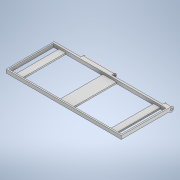
# Autodesk Inventor part: roof
Saved by Autodesk Inventor 2021 (Build 250183000, 183)
## iProperties
Created: 2021-08-17
Part Number: roof
Material: Generisch
Document SubType Name: Modeling
Designer: Tilman
Density: 1 g/cm^3
Appearance: Vorgabe
Author: Tilman
Autodesk Inventor part; units mm, degrees
ref_plane "YZ Plane" through (0, 0, 0) normal (1, 0, 0) x (0, 1, 0)
ref_plane "XZ Plane" through (0, 0, 0) normal (0, 1, 0) x (-1, 0, 0)
ref_plane "XY Plane" through (0, 0, 0) normal (0, 0, 1) x (1, 0, 0)
sketch "Skizze1" plane through (0, 0, 0) normal (0, 1, 0) x (-1, 0, 0)
  line L0 (0, 0) -> (-170, 0)
  line L1 (-170, 0) -> (-170, -70)
  line L2 (-170, -70) -> (0, -70)
  line L3 (0, -70) -> (0, 0)
  dimension "d0" = 170
  dimension "d1" = 70
  constraints: 8 end point, 2 parallel, 1 horizontal, 1 perpendicular
  measures "d0" distance of L0.start L0.end
  measures "d1" distance of L0.end L1.end
extrude "Extrusion1" add sketch "Skizze1" along normal blind 5
sketch "Skizze2" plane through (0, 5, 0) normal (0, 1, 0) x (1, 0, 0)
  line L0 (170, 0) -> (170, 70) projected
  line L1 (170, 70) -> (0, 70) projected
  line L2 (0, 70) -> (0, 0) projected
  line L3 (0, 0) -> (170, 0) projected
  line L4 (2, 68) -> (168, 68)
  line L5 (168, 68) -> (168, 2)
  line L6 (168, 2) -> (2, 2)
  line L7 (2, 2) -> (2, 68)
  dimension "d4" = 2
  constraints: 8 end point, 3 other
  measures "d4" distance between parallel lines of L1 L4
extrude "Extrusion2" cut sketch "Skizze2" against normal blind 3 contours L4 L5 L6 L7
sketch "Skizze3" plane through (0, 2, 0) normal (0, 1, 0) x (1, 0, 0)
  line L0 (168, 2) -> (2, 2) projected
  line L1 (168, 68) -> (168, 2) projected
  line L2 (2, 68) -> (168, 68) projected
  line L3 (2, 2) -> (2, 68) projected
  line L4 (75, 68) -> (95, 68)
  line L5 (95, 68) -> (95, 2)
  line L6 (95, 2) -> (75, 2)
  line L7 (75, 2) -> (75, 68)
  line L8 (2, 68) -> (168, 68) projected
  line L9 (2, 68) -> (168, 68) projected
  line L10 (10, 68) -> (20, 68)
  line L11 (20, 68) -> (20, 2)
  line L12 (20, 2) -> (10, 2)
  line L13 (10, 2) -> (10, 68)
  line L14 (168, 2) -> (2, 2) projected
  line L15 (160, 68) -> (150, 68)
  line L16 (150, 68) -> (150, 2)
  line L17 (150, 2) -> (160, 2)
  line L18 (160, 2) -> (160, 68)
  line L19 (0, 70) -> (0, 0) projected
  line L20 (170, 0) -> (170, 70) projected
  point P0 (85, 68)
  point P1 (85, 68)
  point P2 (160, 2)
  point P3 (10, 2)
  dimension "d7" = 20
  dimension "d8" = 10
  dimension "d9" = 10
  dimension "d10" = 10
  constraints: 24 end point, 6 parallel, 6 point on line, 3 horizontal, 3 perpendicular, 2 midpoint, 1 coincident, 1 collinear
  measures "d7" distance between parallel lines of L5 L7
  measures "d8" distance between parallel lines of L13 L19
  measures "d9" distance between parallel lines of L20 L18
  measures "d10" distance between parallel lines of L18 L16
extrude "Extrusion3" cut sketch "Skizze3" against normal through all contours L0 L18 L2 L1 | L0 L5 L2 L16 | L0 L11 L2 L7 | L0 L3 L2 L13
sketch "Skizze4" plane through (170, 0, 0) normal (1, 0, 0) x (0, 0, -1)
  circle A0 centre (74, 1.5) radius 3.5
  circle A1 centre (74, 1.5) radius 1.75
  line L0 (0, 0) -> (70, 0) projected
  line L1 (0, 5) -> (70, 5) projected
  line L2 (70, 5) -> (74, 5)
  line L3 (70, 0) -> (70, 5) projected
  line L4 (70, 0) -> (70.8377, 0)
  point P0 (70, 3)
  dimension "d13" = 7
  dimension "d14" = 3.5
  dimension "d27" = 4
  constraints: 4 end point, 2 centre point, 2 horizontal, 2 point on circle, 1 coincident, 1 vertical alignment
  measures "d13" diameter of A0
  measures "d14" diameter of A1
  measures "d27" distance from line of L3 A0.centre
extrude "Extrusion4" add sketch "Skizze4" against normal up to surface (170 mm away)
sketch "Skizze5" plane through (0, 5, 0) normal (0, 1, 0) x (1, 0, 0)
  line L0 (170, 70.8377) -> (0, 70.8377) projected
  line L1 (170, 77.5) -> (0, 77.5) projected
  line L2 (170, 70.8377) -> (170, 77.5) projected
  line L3 (0, 70.8377) -> (0, 77.5) projected
  line L4 (170, 77.5) -> (0, 77.5) projected
  line L5 (9.5, 77.5) -> (9.5, 70.8377)
  line L6 (39.5, 70.8377) -> (39.5, 77.5)
  line L7 (160.5, 70.8377) -> (160.5, 77.5)
  line L8 (170, 77.5) -> (0, 77.5) projected
  line L9 (130.5, 70.8377) -> (130.5, 77.5)
  line L10 (85.25, 70.8377) -> (85.25, 77.5)
  line L11 (170, 77.5) -> (0, 77.5) projected
  line L12 (84.75, 77.5) -> (84.75, 70.8377)
  line L13 (85.25, 74.1094) -> (84.75, 74.1094) construction
  point P0 (0, 0)
  point P1 (85, 74.1094)
  point P2 (85, 77.5)
  dimension "d28" = 0.5
  dimension "d29" = 9.5
  dimension "d30" = 9.5
  dimension "d31" = 30
  dimension "d32" = 30
  constraints: 14 end point, 10 point on line, 3 vertical, 2 perpendicular, 1 horizontal, 1 midpoint, 1 parallel, 1 vertical alignment, 7 other
  measures "d28" distance of L13.start L13.end
  measures "d29" distance between parallel lines of L3 L5
  measures "d30" distance between parallel lines of L2 L7
  measures "d31" distance between parallel lines of L7 L9
  measures "d32" distance between parallel lines of L6 L5
extrude "Extrusion5" cut sketch "Skizze5" against normal through all contours L0 L9 L1 L7 | L0 L10 L1 L9 | L0 L5 L1 L6 | L0 L3 L1 L5
equation "\"d9\" = d8"
equation "\"d30\" = d29"
equation "\"d32\" = d31"
